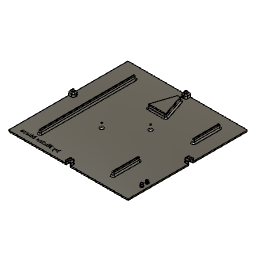
Wordclock_Backplate_Fusion360 (Autodesk Fusion 360 design; units mm, degrees)
Autodesk Fusion 360 part; units mm, degrees
(part 1 of 2)
sketch "Skizze3" plane through (0, 0, 0) normal (0, 0, 1) x (1, 0, 0)
  line L0 (0, 0) -> (204, 0)
  line L1 (204, 0) -> (204, 204)
  line L2 (204, 204) -> (0, 204)
  line L3 (0, 204) -> (0, 0)
  line L4 (2.15, 201.85) -> (201.85, 201.85)
  line L5 (201.85, 201.85) -> (201.85, 2.15)
  line L6 (201.85, 2.15) -> (2.15, 2.15)
  line L7 (2.15, 2.15) -> (2.15, 201.85)
  line L8 (98.5, 204) -> (105.5, 204)
  line L9 (105.5, 204) -> (105.5, 195)
  line L10 (105.5, 195) -> (98.5, 195)
  line L11 (98.5, 195) -> (98.5, 204)
  line L12 (0, 110.5) -> (9, 110.5)
  line L13 (9, 110.5) -> (9, 103.5)
  line L14 (9, 103.5) -> (0, 103.5)
  line L15 (0, 103.5) -> (0, 110.5)
  line L16 (204, 110.5) -> (195, 110.5)
  line L17 (195, 110.5) -> (195, 103.5)
  line L18 (195, 103.5) -> (204, 103.5)
  line L19 (204, 103.5) -> (204, 110.5)
  line L20 (0, 111.5) -> (10, 111.5)
  line L21 (10, 111.5) -> (10, 102.5)
  line L22 (10, 102.5) -> (0, 102.5)
  line L23 (0, 102.5) -> (0, 111.5)
  line L24 (204, 111.5) -> (194, 111.5)
  line L25 (194, 111.5) -> (194, 102.5)
  line L26 (194, 102.5) -> (204, 102.5)
  line L27 (204, 102.5) -> (204, 111.5)
  line L28 (97.5, 204) -> (106.5, 204)
  line L29 (106.5, 204) -> (106.5, 194)
  line L30 (106.5, 194) -> (97.5, 194)
  line L31 (97.5, 194) -> (97.5, 204)
  circle A0 centre (5.5, 107) radius 1.6
  circle A1 centre (102, 198.5) radius 1.6
  circle A2 centre (198.5, 107) radius 1.6
  line L32 (112, 184) -> (92, 184)
  line L33 (92, 184) -> (92, 154)
  line L34 (92, 154) -> (112, 154)
  line L35 (112, 154) -> (112, 184)
  line L36 (112, 154) -> (102, 184)
  line L37 (92, 154) -> (102, 184)
  line L38 (98.5, 0) -> (105.5, 0)
  line L39 (105.5, 0) -> (105.5, 9)
  line L40 (105.5, 9) -> (98.5, 9)
  line L41 (98.5, 9) -> (98.5, 0)
  line L42 (97.5, 0) -> (106.5, 0)
  line L43 (106.5, 0) -> (106.5, 10)
  line L44 (106.5, 10) -> (97.5, 10)
  line L45 (97.5, 10) -> (97.5, 0)
  circle A3 centre (102, 5.5) radius 1.6
  dimension "d16" = 204
  dimension "d17" = 204
  dimension "d18" = 2.15
  dimension "d19" = 2.15
  dimension "d20" = 2.15
  dimension "d21" = 2.15
  dimension "d22" = 7
  dimension "d23" = 9
  dimension "d24" = 98.5
  dimension "d25" = 9
  dimension "d26" = 7
  dimension "d27" = 93.5
  dimension "d28" = 9
  dimension "d29" = 7
  dimension "d30" = 93.5
  dimension "d35" = 1
  dimension "d36" = 1
  dimension "d37" = 1
  dimension "d38" = 1
  dimension "d39" = 1
  dimension "d40" = 1
  dimension "d41" = 1
  dimension "d42" = 1
  dimension "d43" = 1
  dimension "d54" = 3.2
  dimension "d55" = 3.5
  dimension "d56" = 5.5
  dimension "d57" = 3.2
  dimension "d58" = 5.5
  dimension "d59" = 3.5
  dimension "d60" = 3.2
  dimension "d61" = 3.5
  dimension "d62" = 5.5
  dimension "d65" = 20
  dimension "d66" = 30
  dimension "d67" = 20
  dimension "d68" = 92
  dimension "d168" = 7
  dimension "d169" = 9
  dimension "d170" = 98.5
  dimension "d171" = 1
  dimension "d172" = 1
  dimension "d173" = 1
  dimension "d174" = 3.2
  dimension "d175" = 3.5
  dimension "d176" = 5.5
  constraint horizontal L0
  constraint vertical L1
  constraint horizontal L2
  constraint vertical L3
  constraint coincident L0.start L3.end
  constraint horizontal L4
  constraint vertical L5
  constraint horizontal L6
  constraint vertical L7
  constraint horizontal L8
  constraint vertical L9
  constraint horizontal L10
  constraint vertical L11
  constraint coincident L2 L8.start
  constraint horizontal L12
  constraint vertical L13
  constraint horizontal L14
  constraint vertical L15
  constraint coincident L3 L12.start
  constraint horizontal L16
  constraint vertical L17
  constraint horizontal L18
  constraint vertical L19
  constraint coincident L1 L16.start
  constraint horizontal L20
  constraint vertical L21
  constraint horizontal L22
  constraint vertical L23
  constraint coincident L3 L20.start
  constraint horizontal L24
  constraint vertical L25
  constraint horizontal L26
  constraint vertical L27
  constraint coincident L1 L24.start
  constraint horizontal L28
  constraint vertical L29
  constraint horizontal L30
  constraint vertical L31
  constraint coincident L2 L28.start
  constraint horizontal L32
  constraint vertical L33
  constraint horizontal L34
  constraint vertical L35
  constraint midpoint L32 L36.end
  constraint horizontal L38
  constraint vertical L39
  constraint horizontal L40
  constraint vertical L41
  constraint coincident L0 L38.start
  constraint horizontal L42
  constraint vertical L43
  constraint horizontal L44
  constraint vertical L45
  constraint coincident L0 L42.start
  measures "d16" distance of L0.start L2.end
  measures "d17" distance of L0.start L0.end
  measures "d18" distance of L2 L4
  measures "d19" distance of L1 L5
  measures "d20" distance of L3 L7
  measures "d21" distance of L0 L6
  measures "d22" distance of L9.end L10.end
  measures "d23" distance of L8.start L10.end
  measures "d24" distance of L3 L11
  measures "d25" distance of L12.start L12.end
  measures "d26" distance of L12.end L13.end
  measures "d27" distance of L2 L12
  measures "d28" distance of L16.start L16.end
  measures "d29" distance of L16.end L17.end
  measures "d30" distance of L2 L16
  measures "d35" distance of L12 L20
  measures "d36" distance of L14 L22
  measures "d37" distance of L13 L21
  measures "d38" distance of L17 L25
  measures "d39" distance of L16 L24
  measures "d40" distance of L18 L26
  measures "d41" distance of L11 L31
  measures "d42" distance of L10 L30
  measures "d43" distance of L9 L29
  measures "d54" diameter of A0
  measures "d55" distance of L12 A0.centre
  measures "d56" distance of L23 A0.centre
  measures "d57" diameter of A1
  measures "d58" distance of L2 A1.centre
  measures "d59" distance of L9 A1.centre
  measures "d60" diameter of A2
  measures "d61" distance of L16 A2.centre
  measures "d62" distance of L1 A2.centre
  measures "d65" distance of L33.end L34.end
  measures "d66" distance of L32.start L34.end
  measures "d67" distance of L2 L32
  measures "d68" distance of L3 L33
  measures "d168" distance of L39.end L40.end
  measures "d169" distance of L38.start L40.end
  measures "d170" distance of L1 L39
  measures "d171" distance of L40 L44
  measures "d172" distance of L39 L43
  measures "d173" distance of L41 L45
  measures "d174" diameter of A3
  measures "d175" distance of L39 A3.centre
  measures "d176" distance of L0 A3.centre
extrude "Extrusion1" add sketch "Skizze3" along normal blind 2 contours L6 L39 L40 L41 L43 L44 L45 | L4 L5 L6 L7 L20 L21 L22 L24 L25 L26 L29 L30 L31 L43 L44 L45 | L6 L39 L40 L41 | L32 L35 L36 | L32 L33 L37 | L34 L36 L37 | A3
extrude "Extrusion2" add sketch "Skizze3" along normal blind 8 contours L6 L39 L40 L41 L43 L44 L45 | L7 L12 L13 L14 L20 L21 L22 | L6 L39 L40 L41 | L7 L12 L13 L14 | L5 L16 L17 L18 L24 L25 L26 | L4 L9 L10 L11 L29 L30 L31 | L5 L16 L17 L18 | L4 L9 L10 L11 | A0 | A1 | A2 | A3
fillet "Abrundung1" radius 1 4 edges at (201.85, 2.15, 1) (201.85, 201.85, 1) (2.15, 201.85, 1) (2.15, 2.15, 1)
extrude "Extrusion3" cut sketch "Skizze3" along normal blind 6 contours L6 L39 L40 L41 | L7 L12 L13 L14 | L5 L16 L17 L18 | L4 L9 L10 L11 | A0 | A1 | A2 | A3
fillet "Abrundung2" radius 3 8 edges at (194, 102.5, 5) (194, 111.5, 5) (97.5, 194, 5) (106.5, 194, 5) (106.5, 10, 5) (97.5, 10, 5) (10, 111.5, 5) (10, 102.5, 5)
extrude "Extrusion4" cut sketch "Skizze3" along normal blind 8 contours A0 | A1 | A2 | A3
extrude "Extrusion5" cut sketch "Skizze3" along normal blind 3 contours L34 L36 L37
sketch "Skizze4" plane through (0, 0, 2) normal (0, 0, 1) x (-1, 0, 0)
  line L0 (-112, -154) -> (-92, -154)
  line L1 (-92, -154) -> (-102, -184)
  line L2 (-102, -184) -> (-112, -154)
  line L3 (-2.15, -102.5) -> (-2.15, -3.15)
  arc A0 (-2.15, -3.15) -> (-3.15, -2.15) centre (-3.15, -3.15) ccw
  line L4 (-3.15, -2.15) -> (-97.5, -2.15)
  arc A1 (-200.85, -2.15) -> (-201.85, -3.15) centre (-200.85, -3.15) ccw
  line L5 (-201.85, -3.15) -> (-201.85, -102.5)
  arc A2 (-201.85, -200.85) -> (-200.85, -201.85) centre (-200.85, -200.85) ccw
  line L6 (-200.85, -201.85) -> (-106.5, -201.85)
  arc A3 (-3.15, -201.85) -> (-2.15, -200.85) centre (-3.15, -200.85) ccw
  line L7 (-2.15, -200.85) -> (-2.15, -111.5)
  line L8 (-89.2251, -152) -> (-115.201, -152)
  line L9 (-89.2147, -151.9686) -> (-100.633, -186.2236)
  line L10 (-103.3833, -186.1747) -> (-114.7974, -151.9325)
  line L11 (-104.7948, -188.2647) -> (-117.816, -149.2012)
  line L12 (-86.4032, -149.8589) -> (-99.2936, -188.5299)
  line L13 (-86, -150) -> (-118, -150)
  line L14 (-104, -186) -> (-100, -186)
  line L15 (-105.9099, -187.9999) -> (-98.0331, -188.0001)
  line L16 (-97.5, -2.15) -> (-97.5, -7)
  arc A4 (-100.5, -10) -> (-97.5, -7) centre (-100.5, -7) ccw
  line L17 (-100.5, -10) -> (-103.5, -10)
  arc A5 (-106.5, -7) -> (-103.5, -10) centre (-103.5, -7) ccw
  line L18 (-106.5, -7) -> (-106.5, -2.15)
  line L19 (-106.5, -2.15) -> (-200.85, -2.15)
  line L20 (-201.85, -102.5) -> (-197, -102.5)
  arc A6 (-194, -105.5) -> (-197, -102.5) centre (-197, -105.5) ccw
  line L21 (-194, -105.5) -> (-194, -108.5)
  arc A7 (-197, -111.5) -> (-194, -108.5) centre (-197, -108.5) ccw
  line L22 (-197, -111.5) -> (-201.85, -111.5)
  line L23 (-201.85, -111.5) -> (-201.85, -200.85)
  line L24 (-106.5, -201.85) -> (-106.5, -197)
  arc A8 (-103.5, -194) -> (-106.5, -197) centre (-103.5, -197) ccw
  line L25 (-103.5, -194) -> (-100.5, -194)
  arc A9 (-97.5, -197) -> (-100.5, -194) centre (-100.5, -197) ccw
  line L26 (-97.5, -197) -> (-97.5, -201.85)
  line L27 (-97.5, -201.85) -> (-3.15, -201.85)
  line L28 (-2.15, -111.5) -> (-7, -111.5)
  arc A10 (-10, -108.5) -> (-7, -111.5) centre (-7, -108.5) ccw
  line L29 (-10, -108.5) -> (-10, -105.5)
  arc A11 (-7, -102.5) -> (-10, -105.5) centre (-7, -105.5) ccw
  line L30 (-7, -102.5) -> (-2.15, -102.5)
  dimension "d75" = 2
  dimension "d78" = 2
  dimension "d79" = 2
  dimension "d84" = 2
  dimension "d85" = 2
  dimension "d86" = 2
  dimension "d87" = 2
  dimension "d88" = 2
  constraint horizontal L8
  constraint coincident L8.start L9
  constraint horizontal L13
  measures "d75" distance of L0 L8
  measures "d78" distance of L1 L9
  measures "d79" distance of L2 L10
  measures "d84" distance of L10 L11
  measures "d85" distance of L9 L12
  measures "d86" distance of L8 L13
  measures "d87" distance of L1.end L14
  measures "d88" distance of L14 L15
extrude "Extrusion8" add sketch "Skizze4" along normal blind 6.25 contours L11 L12 L13 L15
sketch "Skizze6" plane through (0, 0, 8.25) normal (0, 0, 1) x (-1, 0, 0)
  line L0 (-114.7749, -152) -> (-89.2251, -152)
  line L1 (-89.2251, -152) -> (-100.5585, -186)
  line L2 (-100.5585, -186) -> (-103.4415, -186)
  line L3 (-103.4415, -186) -> (-114.7749, -152)
  line L4 (-86.4503, -150) -> (-117.5497, -150)
  line L5 (-117.5497, -150) -> (-104.8831, -188)
  line L6 (-104.8831, -188) -> (-99.117, -188)
  line L7 (-99.117, -188) -> (-86.4503, -150)
extrude "Extrusion9" add sketch "Skizze6" against normal blind 2 contours L0 L1 L2 L3
fillet "Abrundung3" radius 2 3 edges at (102, 184, 1) (112, 154, 1) (92, 154, 1)
sketch "Skizze7" plane through (0, 0, 2) normal (0, 0, 1) x (-1, 0, 0)
  line L0 (-2.15, -102.5) -> (-2.15, -3.15)
  arc A0 (-2.15, -3.15) -> (-3.15, -2.15) centre (-3.15, -3.15) ccw
  line L1 (-3.15, -2.15) -> (-97.5, -2.15)
  arc A1 (-200.85, -2.15) -> (-201.85, -3.15) centre (-200.85, -3.15) ccw
  line L2 (-201.85, -3.15) -> (-201.85, -102.5)
  arc A2 (-201.85, -200.85) -> (-200.85, -201.85) centre (-200.85, -200.85) ccw
  line L3 (-200.85, -201.85) -> (-106.5, -201.85)
  arc A3 (-3.15, -201.85) -> (-2.15, -200.85) centre (-3.15, -200.85) ccw
  line L4 (-2.15, -200.85) -> (-2.15, -111.5)
  line L5 (-86.4503, -150) -> (-99.117, -188)
  line L6 (-99.117, -188) -> (-104.8831, -188)
  line L7 (-104.8831, -188) -> (-117.5497, -150)
  line L8 (-117.5497, -150) -> (-86.4503, -150)
  circle A4 centre (-77, -83) radius 1.25
  circle A5 centre (-120.538, -121.321) radius 1.25
  line L9 (-97.5, -2.15) -> (-97.5, -7)
  arc A6 (-100.5, -10) -> (-97.5, -7) centre (-100.5, -7) ccw
  line L10 (-100.5, -10) -> (-103.5, -10)
  arc A7 (-106.5, -7) -> (-103.5, -10) centre (-103.5, -7) ccw
  line L11 (-106.5, -7) -> (-106.5, -2.15)
  line L12 (-106.5, -2.15) -> (-200.85, -2.15)
  line L13 (-201.85, -102.5) -> (-197, -102.5)
  arc A8 (-194, -105.5) -> (-197, -102.5) centre (-197, -105.5) ccw
  line L14 (-194, -105.5) -> (-194, -108.5)
  arc A9 (-197, -111.5) -> (-194, -108.5) centre (-197, -108.5) ccw
  line L15 (-197, -111.5) -> (-201.85, -111.5)
  line L16 (-201.85, -111.5) -> (-201.85, -200.85)
  line L17 (-106.5, -201.85) -> (-106.5, -197)
  arc A10 (-103.5, -194) -> (-106.5, -197) centre (-103.5, -197) ccw
  line L18 (-103.5, -194) -> (-100.5, -194)
  arc A11 (-97.5, -197) -> (-100.5, -194) centre (-100.5, -197) ccw
  line L19 (-97.5, -197) -> (-97.5, -201.85)
  line L20 (-97.5, -201.85) -> (-3.15, -201.85)
  line L21 (-2.15, -111.5) -> (-7, -111.5)
  arc A12 (-10, -108.5) -> (-7, -111.5) centre (-7, -108.5) ccw
  line L22 (-10, -108.5) -> (-10, -105.5)
  arc A13 (-7, -102.5) -> (-10, -105.5) centre (-7, -105.5) ccw
  line L23 (-7, -102.5) -> (-2.15, -102.5)
  dimension "d95" = 2.5
  dimension "d97" = 74.85
  dimension "d98" = 2.5
  dimension "d99" = 80.529
  measures "d95" diameter of A4
  measures "d97" distance of L0 A4.centre
  measures "d98" diameter of A5
  measures "d99" distance of L3 A5.centre
extrude "Extrusion10" add sketch "Skizze7" along normal blind 8 contours A4 | A5
fillet "Abrundung4" radius 2 2 edges at (78.1654, 82.548, 2) (121.7034, 120.869, 2)
sketch "Skizze8" plane through (0, 0, 2) normal (0, 0, 1) x (-1, 0, 0)
  circle A0 centre (-77, -83) radius 3.25
  line L0 (-2.15, -102.5) -> (-2.15, -3.15)
  arc A1 (-2.15, -3.15) -> (-3.15, -2.15) centre (-3.15, -3.15) ccw
  line L1 (-3.15, -2.15) -> (-97.5, -2.15)
  arc A2 (-200.85, -2.15) -> (-201.85, -3.15) centre (-200.85, -3.15) ccw
  line L2 (-201.85, -3.15) -> (-201.85, -102.5)
  arc A3 (-201.85, -200.85) -> (-200.85, -201.85) centre (-200.85, -200.85) ccw
  line L3 (-200.85, -201.85) -> (-106.5, -201.85)
  arc A4 (-3.15, -201.85) -> (-2.15, -200.85) centre (-3.15, -200.85) ccw
  line L4 (-2.15, -200.85) -> (-2.15, -111.5)
  line L5 (-86.4503, -150) -> (-99.117, -188)
  line L6 (-99.117, -188) -> (-104.8831, -188)
  line L7 (-104.8831, -188) -> (-117.5497, -150)
  line L8 (-117.5497, -150) -> (-86.4503, -150)
  circle A5 centre (-120.538, -121.321) radius 3.25
  circle A6 centre (-194.85, -32.15) radius 2.5
  circle A7 centre (-194.85, -32.15) radius 1.5
  circle A8 centre (-194.85, -41.15) radius 2.5
  circle A9 centre (-194.85, -41.15) radius 1.5
  line L9 (-97.5, -2.15) -> (-97.5, -7)
  arc A10 (-100.5, -10) -> (-97.5, -7) centre (-100.5, -7) ccw
  line L10 (-100.5, -10) -> (-103.5, -10)
  arc A11 (-106.5, -7) -> (-103.5, -10) centre (-103.5, -7) ccw
  line L11 (-106.5, -7) -> (-106.5, -2.15)
  line L12 (-106.5, -2.15) -> (-200.85, -2.15)
  line L13 (-201.85, -102.5) -> (-197, -102.5)
  arc A12 (-194, -105.5) -> (-197, -102.5) centre (-197, -105.5) ccw
  line L14 (-194, -105.5) -> (-194, -108.5)
  arc A13 (-197, -111.5) -> (-194, -108.5) centre (-197, -108.5) ccw
  line L15 (-197, -111.5) -> (-201.85, -111.5)
  line L16 (-201.85, -111.5) -> (-201.85, -200.85)
  line L17 (-106.5, -201.85) -> (-106.5, -197)
  arc A14 (-103.5, -194) -> (-106.5, -197) centre (-103.5, -197) ccw
  line L18 (-103.5, -194) -> (-100.5, -194)
  arc A15 (-97.5, -197) -> (-100.5, -194) centre (-100.5, -197) ccw
  line L19 (-97.5, -197) -> (-97.5, -201.85)
  line L20 (-97.5, -201.85) -> (-3.15, -201.85)
  line L21 (-2.15, -111.5) -> (-7, -111.5)
  arc A16 (-10, -108.5) -> (-7, -111.5) centre (-7, -108.5) ccw
  line L22 (-10, -108.5) -> (-10, -105.5)
  arc A17 (-7, -102.5) -> (-10, -105.5) centre (-7, -105.5) ccw
  line L23 (-7, -102.5) -> (-2.15, -102.5)
  dimension "d105" = 5
  dimension "d106" = 7
  dimension "d107" = 30
  dimension "d108" = 3
  dimension "d109" = 5
  dimension "d110" = 3
  dimension "d111" = 7
  dimension "d112" = 9
  constraint concentric A6 A7
  constraint concentric A8 A9
  measures "d105" diameter of A6
  measures "d106" distance of L2 A6.centre
  measures "d107" distance of L1 A6.centre
  measures "d108" diameter of A7
  measures "d109" diameter of A8
  measures "d110" diameter of A9
  measures "d111" distance of L2 A8.centre
  measures "d112" distance of A6.centre A8.centre
extrude "Extrusion11" add sketch "Skizze8" along normal blind 1 contours A6 | A8
extrude "Extrusion12" add sketch "Skizze8" along normal blind 3.5 contours A7 | A9
sketch "Skizze9" plane through (0, 0, 5.5) normal (0, 0, 1) x (-1, 0, 0)
  circle A0 centre (-194.85, -41.15) radius 1.5
  circle A1 centre (-194.85, -41.15) radius 2
  circle A2 centre (-194.85, -32.15) radius 1.5
  circle A3 centre (-194.85, -32.15) radius 2
  dimension "d117" = 4
  dimension "d119" = 4
  constraint concentric A0 A1
  constraint concentric A2 A3
  measures "d117" diameter of A1
  measures "d119" diameter of A3
extrude "Extrusion13" add sketch "Skizze9" along normal blind 2 contours A0 | A1 | A2 | A3
sketch "Skizze10" plane through (0, 0, 7.5) normal (0, 0, 1) x (-1, 0, 0)
  circle A0 centre (-194.85, -41.15) radius 2
  line L0 (-193.1, -42.9) -> (-196.6, -42.9)
  line L1 (-196.6, -42.9) -> (-196.6, -39.4)
  line L2 (-196.6, -39.4) -> (-193.1, -39.4)
  line L3 (-193.1, -39.4) -> (-193.1, -42.9)
  line L4 (-193.1, -42.9) -> (-196.6, -39.4)
  line L5 (-192.7464, -42.5464) -> (-196.2464, -39.0464)
  line L6 (-193.4667, -43.2404) -> (-196.9667, -39.7404)
  line L7 (-193.1, -30.4) -> (-193.1, -33.9)
  line L8 (-192.7596, -30.7667) -> (-196.2596, -34.2667)
  line L9 (-193.1, -30.4) -> (-196.6, -33.9)
  line L10 (-193.4536, -30.0464) -> (-196.9536, -33.5464)
  line L11 (-196.6, -30.4) -> (-193.1, -30.4)
  line L12 (-196.6, -33.9) -> (-196.6, -30.4)
  line L13 (-193.1, -33.9) -> (-196.6, -33.9)
  dimension "d122" = 1.75
  dimension "d123" = 3.5
  dimension "d124" = 1.75
  dimension "d125" = 3.5
  dimension "d127" = 1
  dimension "d128" = 0.5
  dimension "d129" = 3.5
  dimension "d130" = 3.5
  dimension "d131" = 1
  dimension "d132" = 0.5
  constraint horizontal L0
  constraint vertical L1
  constraint horizontal L2
  constraint vertical L3
  measures "d122" distance of A0.centre L3
  measures "d123" distance of L1 L3
  measures "d124" distance of A0.centre L0
  measures "d125" distance of L0.end L1.end
  measures "d127" distance of L5 L6
  measures "d128" distance of L4 L5
  measures "d129" distance of L11 L13
  measures "d130" distance of L7.end L9.end
  measures "d131" distance of L8 L10
  measures "d132" distance of L9 L10
chamfer "Fase1" distance 1.5 angle 45 2 edges at (196.7147, 41.8732, 7.5) (196.7147, 32.8732, 7.5)
extrude "Extrusion14" cut sketch "Skizze10" against normal blind 5 contours A0 L3 L4 L5 | A0 L4 L5 | A0 L0 L4 L6 | A0 L4 L6 | A0 L2 L4 L5 | A0 L1 L4 L6 | L7 L8 L9 L13 | L9 L10 L11 L12
fillet "Abrundung10" radius 3 8 edges at (98.5, 195, 3) (105.5, 195, 3) (9, 103.5, 3) (9, 110.5, 3) (105.5, 9, 3) (98.5, 9, 3) (195, 110.5, 3) (195, 103.5, 3)
fillet "Abrundung11" radius 2 20 edges at (4.575, 102.5, 8) (9.1213, 103.3787, 8) (10, 107, 8) (9.1213, 110.6213, 8) (4.575, 111.5, 8) (106.5, 199.425, 8) (105.6213, 194.8787, 8) (102, 194, 8) (98.3787, 194.8787, 8) (97.5, 199.425, 8) (199.425, 102.5, 8) (194.8787, 103.3787, 8) (194, 107, 8) (194.8787, 110.6213, 8) (199.425, 111.5, 8) (106.5, 4.575, 8) (105.6213, 9.1213, 8) (102, 10, 8) (98.3787, 9.1213, 8) (97.5, 4.575, 8)
sketch "Skizze11" plane through (0, 0, 2) normal (0, 0, 1) x (-1, 0, 0)
  circle A0 centre (-194.85, -41.15) radius 2.5
  circle A1 centre (-77, -83) radius 3.25
  line L0 (-2.15, -102.5) -> (-2.15, -3.15)
  arc A2 (-2.15, -3.15) -> (-3.15, -2.15) centre (-3.15, -3.15) ccw
  line L1 (-3.15, -2.15) -> (-97.5, -2.15)
  arc A3 (-200.85, -2.15) -> (-201.85, -3.15) centre (-200.85, -3.15) ccw
  line L2 (-201.85, -3.15) -> (-201.85, -102.5)
  arc A4 (-201.85, -200.85) -> (-200.85, -201.85) centre (-200.85, -200.85) ccw
  line L3 (-200.85, -201.85) -> (-106.5, -201.85)
  arc A5 (-3.15, -201.85) -> (-2.15, -200.85) centre (-3.15, -200.85) ccw
  line L4 (-2.15, -200.85) -> (-2.15, -111.5)
  line L5 (-86.4503, -150) -> (-99.117, -188)
  line L6 (-99.117, -188) -> (-104.8831, -188)
  line L7 (-104.8831, -188) -> (-117.5497, -150)
  line L8 (-117.5497, -150) -> (-86.4503, -150)
  circle A6 centre (-120.538, -121.321) radius 3.25
  circle A7 centre (-194.85, -32.15) radius 2.5
  line L9 (-32.15, -181.85) -> (-35.15, -181.85)
  line L10 (-35.15, -181.85) -> (-35.15, -22.15)
  line L11 (-35.15, -22.15) -> (-32.15, -22.15)
  line L12 (-32.15, -22.15) -> (-32.15, -181.85)
  line L13 (-173.85, -181.85) -> (-176.85, -181.85)
  line L14 (-176.85, -181.85) -> (-176.85, -136.85)
  line L15 (-176.85, -136.85) -> (-173.85, -136.85)
  line L16 (-173.85, -136.85) -> (-173.85, -181.85)
  line L17 (-153.85, -67.15) -> (-156.85, -67.15)
  line L18 (-156.85, -67.15) -> (-156.85, -22.15)
  line L19 (-156.85, -22.15) -> (-153.85, -22.15)
  line L20 (-153.85, -22.15) -> (-153.85, -67.15)
  line L21 (-97.5, -2.15) -> (-97.5, -7)
  arc A8 (-100.5, -10) -> (-97.5, -7) centre (-100.5, -7) ccw
  line L22 (-100.5, -10) -> (-103.5, -10)
  arc A9 (-106.5, -7) -> (-103.5, -10) centre (-103.5, -7) ccw
  line L23 (-106.5, -7) -> (-106.5, -2.15)
  line L24 (-106.5, -2.15) -> (-200.85, -2.15)
  line L25 (-201.85, -102.5) -> (-197, -102.5)
  arc A10 (-194, -105.5) -> (-197, -102.5) centre (-197, -105.5) ccw
  line L26 (-194, -105.5) -> (-194, -108.5)
  arc A11 (-197, -111.5) -> (-194, -108.5) centre (-197, -108.5) ccw
  line L27 (-197, -111.5) -> (-201.85, -111.5)
  line L28 (-201.85, -111.5) -> (-201.85, -200.85)
  line L29 (-106.5, -201.85) -> (-106.5, -197)
  arc A12 (-103.5, -194) -> (-106.5, -197) centre (-103.5, -197) ccw
  line L30 (-103.5, -194) -> (-100.5, -194)
  arc A13 (-97.5, -197) -> (-100.5, -194) centre (-100.5, -197) ccw
  line L31 (-97.5, -197) -> (-97.5, -201.85)
  line L32 (-97.5, -201.85) -> (-3.15, -201.85)
  line L33 (-2.15, -111.5) -> (-7, -111.5)
  arc A14 (-10, -108.5) -> (-7, -111.5) centre (-7, -108.5) ccw
  line L34 (-10, -108.5) -> (-10, -105.5)
  arc A15 (-7, -102.5) -> (-10, -105.5) centre (-7, -105.5) ccw
  line L35 (-7, -102.5) -> (-2.15, -102.5)
  dimension "d136" = 3
  dimension "d138" = 20
  dimension "d139" = 20
  dimension "d145" = 45
  dimension "d147" = 3
  dimension "d149" = 3
  dimension "d150" = 45
  dimension "d151" = 20
  dimension "d152" = 30
  dimension "d154" = 45
  dimension "d181" = 25
  constraint horizontal L9
  constraint vertical L10
  constraint horizontal L11
  constraint vertical L12
  constraint horizontal L13
  constraint vertical L14
  constraint horizontal L15
  constraint vertical L16
  constraint horizontal L17
  constraint vertical L18
  constraint horizontal L19
  constraint vertical L20
  measures "d136" distance of L10 L12
  measures "d138" distance of L3 L9
  measures "d139" distance of L1 L11
  measures "d145" distance of L13.end L14.end
  measures "d147" distance of L13.start L13.end
  measures "d149" distance of L17.start L17.end
  measures "d150" distance of L17.end L18.end
  measures "d151" distance of L1 L19
  measures "d152" distance of L4 L12
  measures "d154" distance of L2 L18
  measures "d181" distance of L14 L28
extrude "Extrusion16" add sketch "Skizze11" along normal blind 6.25 contours L9 L10 L11 L12 | L13 L14 L15 L16 | L17 L18 L19 L20
sketch "Skizze12" plane through (0, 0, 0) normal (0, 0, -1) x (1, 0, 0)
  line L0 (94.7749, -154) -> (109.2251, -154)
  arc A0 (111.1225, -156.6325) -> (109.2251, -154) centre (109.2251, -156) ccw
  line L1 (111.1225, -156.6325) -> (103.8974, -178.3079)
  arc A1 (100.1026, -178.3079) -> (103.8974, -178.3079) centre (102, -177.6754) ccw
  line L2 (100.1026, -178.3079) -> (92.8775, -156.6325)
  arc A2 (94.7749, -154) -> (92.8775, -156.6325) centre (94.7749, -156) ccw
  line L3 (6, -110.5) -> (2.15, -110.5)
  line L4 (2.15, -110.5) -> (2.15, -200.85)
  arc A3 (2.15, -200.85) -> (3.15, -201.85) centre (3.15, -200.85) ccw
  line L5 (3.15, -201.85) -> (98.5, -201.85)
  line L6 (98.5, -201.85) -> (98.5, -198)
  line L7 (101.5, -195) -> (102.5, -195)
  line L8 (105.5, -198) -> (105.5, -201.85)
  line L9 (105.5, -201.85) -> (200.85, -201.85)
  arc A4 (200.85, -201.85) -> (201.85, -200.85) centre (200.85, -200.85) ccw
  line L10 (201.85, -200.85) -> (201.85, -110.5)
  line L11 (201.85, -110.5) -> (198, -110.5)
  line L12 (195, -107.5) -> (195, -106.5)
  line L13 (198, -103.5) -> (201.85, -103.5)
  line L14 (201.85, -103.5) -> (201.85, -3.15)
  arc A5 (201.85, -3.15) -> (200.85, -2.15) centre (200.85, -3.15) ccw
  line L15 (200.85, -2.15) -> (105.5, -2.15)
  arc A6 (3.15, -2.15) -> (2.15, -3.15) centre (3.15, -3.15) ccw
  line L16 (2.15, -3.15) -> (2.15, -103.5)
  line L17 (2.15, -103.5) -> (6, -103.5)
  line L18 (9, -106.5) -> (9, -107.5)
  line L19 (75.219, -11.0615) -> (75.219, -11.7939)
  line L20 (75.219, -11.7939) -> (74.4736, -11.7939)
  line L21 (74.4736, -11.7939) -> (74.4736, -16.3578)
  line L22 (74.4736, -16.3578) -> (75.219, -16.3578)
  line L23 (75.219, -16.3578) -> (75.219, -17.0903)
  line L24 (75.219, -17.0903) -> (73.6674, -17.0903)
  line L25 (73.6674, -17.0903) -> (73.6674, -14.6631)
  spline S0 degree 2 poles (73.6674, -14.6631) (73.0476, -15.3739) (72.1461, -15.3739) knots 0 0 0 1 1 1
  spline S1 degree 2 poles (72.1461, -15.3739) (71.2793, -15.3739) (70.6942, -14.7758) knots 0 0 0 1 1 1
  spline S2 degree 2 poles (70.6942, -14.7758) (70.1047, -14.1821) (70.1047, -13.2069) knots 0 0 0 1 1 1
  spline S3 degree 2 poles (70.1047, -13.2069) (70.1047, -12.2707) (70.6812, -11.6292) knots 0 0 0 1 1 1
  spline S4 degree 2 poles (70.6812, -11.6292) (71.2533, -10.9921) (72.1504, -10.9921) knots 0 0 0 1 1 1
  spline S5 degree 2 poles (72.1504, -10.9921) (72.6532, -10.9921) (73.0693, -11.2088) knots 0 0 0 1 1 1
  spline S6 degree 2 poles (73.0693, -11.2088) (73.4854, -11.4255) (73.6674, -11.6899) knots 0 0 0 1 1 1
  line L26 (73.6674, -11.6899) -> (73.6674, -11.0615)
  line L27 (73.6674, -11.0615) -> (75.219, -11.0615)
  spline S7 degree 2 poles (73.6414, -13.1505) (73.6414, -12.4961) (73.2426, -12.1103) knots 0 0 0 1 1 1
  spline S8 degree 2 poles (73.2426, -12.1103) (72.8396, -11.7289) (72.3151, -11.7289) knots 0 0 0 1 1 1
  spline S9 degree 2 poles (72.3151, -11.7289) (71.7647, -11.7289) (71.366, -12.1363) knots 0 0 0 1 1 1
  spline S10 degree 2 poles (71.366, -12.1363) (70.9672, -12.5437) (70.9672, -13.2285) knots 0 0 0 1 1 1
  spline S11 degree 2 poles (70.9672, -13.2285) (70.9672, -13.8917) (71.366, -14.2557) knots 0 0 0 1 1 1
  spline S12 degree 2 poles (71.366, -14.2557) (71.7604, -14.6241) (72.2935, -14.6241) knots 0 0 0 1 1 1
  spline S13 degree 2 poles (72.2935, -14.6241) (72.8179, -14.6241) (73.2296, -14.2427) knots 0 0 0 1 1 1
  spline S14 degree 2 poles (73.2296, -14.2427) (73.6414, -13.8657) (73.6414, -13.1505) knots 0 0 0 1 1 1
  line L28 (67.916, -11.1351) -> (69.2942, -14.5244)
  line L29 (69.2942, -14.5244) -> (69.992, -14.5244)
  line L30 (69.992, -14.5244) -> (69.992, -15.2569)
  line L31 (69.992, -15.2569) -> (67.916, -15.2569)
  line L32 (67.916, -15.2569) -> (67.916, -14.5244)
  line L33 (67.916, -14.5244) -> (68.4187, -14.5244)
  line L34 (68.4187, -14.5244) -> (67.5129, -12.2013)
  line L35 (67.5129, -12.2013) -> (66.6244, -14.5244)
  line L36 (66.6244, -14.5244) -> (67.1792, -14.5244)
  line L37 (67.1792, -14.5244) -> (67.1792, -15.2569)
  line L38 (67.1792, -15.2569) -> (65.1464, -15.2569)
  line L39 (65.1464, -15.2569) -> (65.1464, -14.5244)
  line L40 (65.1464, -14.5244) -> (65.7706, -14.5244)
  line L41 (65.7706, -14.5244) -> (67.8466, -9.1804)
  line L42 (67.8466, -9.1804) -> (69.2379, -9.1804)
  line L43 (69.2379, -9.1804) -> (69.2379, -9.8999)
  line L44 (69.2379, -9.8999) -> (68.4187, -9.8999)
  line L45 (68.4187, -9.8999) -> (67.916, -11.1351)
  line L46 (61.9435, -11.8156) -> (61.9435, -16.3361)
  line L47 (61.9435, -16.3361) -> (62.806, -16.3361)
  line L48 (62.806, -16.3361) -> (62.806, -17.0903)
  line L49 (62.806, -17.0903) -> (60.7473, -17.0903)
  line L50 (60.7473, -17.0903) -> (58.1034, -12.405)
  line L51 (58.1034, -12.405) -> (58.1034, -16.3361)
  line L52 (58.1034, -16.3361) -> (58.9573, -16.3361)
  line L53 (58.9573, -16.3361) -> (58.9573, -17.0903)
  line L54 (58.9573, -17.0903) -> (56.4825, -17.0903)
  line L55 (56.4825, -17.0903) -> (56.4825, -16.3361)
  line L56 (56.4825, -16.3361) -> (57.371, -16.3361)
  line L57 (57.371, -16.3361) -> (57.371, -11.0008)
  line L58 (57.371, -11.0008) -> (58.3072, -11.0008)
  line L59 (58.3072, -11.0008) -> (61.198, -16.1454)
  line L60 (61.198, -16.1454) -> (61.198, -11.8156)
  line L61 (61.198, -11.8156) -> (60.3355, -11.8156)
  line L62 (60.3355, -11.8156) -> (60.3355, -11.0614)
  line L63 (60.3355, -11.0614) -> (62.806, -11.0614)
  line L64 (62.806, -11.0614) -> (62.806, -11.8156)
  line L65 (62.806, -11.8156) -> (61.9435, -11.8156)
  spline S15 degree 2 poles (55.646, -16.6829) (55.646, -16.8822) (55.5073, -17.0296) knots 0 0 0 1 1 1
  spline S16 degree 2 poles (55.5073, -17.0296) (55.3643, -17.1769) (55.1476, -17.1769) knots 0 0 0 1 1 1
  spline S17 degree 2 poles (55.1476, -17.1769) (54.9438, -17.1769) (54.7965, -17.0339) knots 0 0 0 1 1 1
  spline S18 degree 2 poles (54.7965, -17.0339) (54.6491, -16.8909) (54.6491, -16.6829) knots 0 0 0 1 1 1
  spline S19 degree 2 poles (54.6491, -16.6829) (54.6491, -16.4748) (54.7965, -16.3275) knots 0 0 0 1 1 1
  spline S20 degree 2 poles (54.7965, -16.3275) (54.9438, -16.1844) (55.1476, -16.1844) knots 0 0 0 1 1 1
  spline S21 degree 2 poles (55.1476, -16.1844) (55.3556, -16.1844) (55.503, -16.3318) knots 0 0 0 1 1 1
  spline S22 degree 2 poles (55.503, -16.3318) (55.646, -16.4791) (55.646, -16.6829) knots 0 0 0 1 1 1
  line L66 (55.529, -11.7939) -> (55.529, -14.5244)
  line L67 (55.529, -14.5244) -> (56.1834, -14.5244)
  line L68 (56.1834, -14.5244) -> (56.1834, -15.2569)
  line L69 (56.1834, -15.2569) -> (54.7055, -15.2569)
  line L70 (54.7055, -15.2569) -> (54.7055, -11.7939)
  line L71 (54.7055, -11.7939) -> (54.0597, -11.7939)
  line L72 (54.0597, -11.7939) -> (54.0597, -11.0615)
  line L73 (54.0597, -11.0615) -> (56.1834, -11.0615)
  line L74 (56.1834, -11.0615) -> (56.1834, -11.7939)
  line L75 (56.1834, -11.7939) -> (55.529, -11.7939)
  line L76 (49.5782, -15.2569) -> (49.5782, -13.6706)
  line L77 (49.5782, -13.6706) -> (50.315, -13.6706)
  spline S23 degree 2 poles (50.315, -13.6706) (50.3713, -14.1257) (50.6877, -14.3684) knots 0 0 0 1 1 1
  spline S24 degree 2 poles (50.6877, -14.3684) (50.9998, -14.6111) (51.4158, -14.6111) knots 0 0 0 1 1 1
  spline S25 degree 2 poles (51.4158, -14.6111) (51.9706, -14.6111) (52.3174, -14.2167) knots 0 0 0 1 1 1
  spline S26 degree 2 poles (52.3174, -14.2167) (52.6641, -13.8267) (52.6641, -13.1895) knots 0 0 0 1 1 1
  spline S27 degree 2 poles (52.6641, -13.1895) (52.6641, -12.5958) (52.3347, -12.1407) knots 0 0 0 1 1 1
  spline S28 degree 2 poles (52.3347, -12.1407) (52.0053, -11.6899) (51.3812, -11.6899) knots 0 0 0 1 1 1
  spline S29 degree 2 poles (51.3812, -11.6899) (50.5143, -11.6899) (50.1243, -12.5134) knots 0 0 0 1 1 1
  line L78 (50.1243, -12.5134) -> (49.4438, -12.1927)
  spline S30 degree 2 poles (49.4438, -12.1927) (50.0072, -10.9401) (51.4158, -10.9401) knots 0 0 0 1 1 1
  spline S31 degree 2 poles (51.4158, -10.9401) (52.4127, -10.9401) (52.9848, -11.6206) knots 0 0 0 1 1 1
  spline S32 degree 2 poles (52.9848, -11.6206) (53.5569, -12.301) (53.5569, -13.1895) knots 0 0 0 1 1 1
  spline S33 degree 2 poles (53.5569, -13.1895) (53.5569, -14.1387) (52.9328, -14.7542) knots 0 0 0 1 1 1
  spline S34 degree 2 poles (52.9328, -14.7542) (52.3087, -15.3739) (51.4939, -15.3739) knots 0 0 0 1 1 1
  spline S35 degree 2 poles (51.4939, -15.3739) (50.7961, -15.3739) (50.315, -14.9622) knots 0 0 0 1 1 1
  line L79 (50.315, -14.9622) -> (50.315, -15.2569)
  line L80 (50.315, -15.2569) -> (49.5782, -15.2569)
  line L81 (48.3169, -11.7939) -> (48.3169, -16.3578)
  line L82 (48.3169, -16.3578) -> (49.0624, -16.3578)
  line L83 (49.0624, -16.3578) -> (49.0624, -17.0903)
  line L84 (49.0624, -17.0903) -> (47.4934, -17.0903)
  line L85 (47.4934, -17.0903) -> (47.4934, -11.7939)
  line L86 (47.4934, -11.7939) -> (46.852, -11.7939)
  line L87 (46.852, -11.7939) -> (46.852, -11.0615)
  line L88 (46.852, -11.0615) -> (49.0624, -11.0615)
  line L89 (49.0624, -11.0615) -> (49.0624, -11.7939)
  line L90 (49.0624, -11.7939) -> (48.3169, -11.7939)
  line L91 (42.0411, -11.7939) -> (42.0411, -11.0615)
  line L92 (42.0411, -11.0615) -> (43.48, -11.0615)
  line L93 (43.48, -11.0615) -> (43.48, -11.5729)
  spline S36 degree 2 poles (43.48, -11.5729) (44.0781, -10.9921) (44.8149, -10.9921) knots 0 0 0 1 1 1
  spline S37 degree 2 poles (44.8149, -10.9921) (45.387, -10.9921) (45.8118, -11.3648) knots 0 0 0 1 1 1
  spline S38 degree 2 poles (45.8118, -11.3648) (46.2322, -11.7376) (46.2322, -12.3184) knots 0 0 0 1 1 1
  spline S39 degree 2 poles (46.2322, -12.3184) (46.2322, -12.9035) (45.7858, -13.2892) knots 0 0 0 1 1 1
  spline S40 degree 2 poles (45.7858, -13.2892) (45.335, -13.675) (44.7022, -13.675) knots 0 0 0 1 1 1
  spline S41 degree 2 poles (44.7022, -13.675) (44.1128, -13.675) (43.5624, -13.3196) knots 0 0 0 1 1 1
  line L94 (43.5624, -13.3196) -> (43.5624, -13.7356)
  spline S42 degree 2 poles (43.5624, -13.7356) (43.5624, -14.0564) (43.623, -14.2297) knots 0 0 0 1 1 1
  spline S43 degree 2 poles (43.623, -14.2297) (43.6837, -14.4031) (43.9091, -14.5418) knots 0 0 0 1 1 1
  spline S44 degree 2 poles (43.9091, -14.5418) (44.1301, -14.6805) (44.4898, -14.6805) knots 0 0 0 1 1 1
  spline S45 degree 2 poles (44.4898, -14.6805) (45.1096, -14.6805) (45.387, -14.1864) knots 0 0 0 1 1 1
  line L95 (45.387, -14.1864) -> (46.1758, -14.3944)
  spline S46 degree 2 poles (46.1758, -14.3944) (45.6514, -15.3739) (44.3642, -15.3739) knots 0 0 0 1 1 1
  spline S47 degree 2 poles (44.3642, -15.3739) (43.8917, -15.3739) (43.5493, -15.2439) knots 0 0 0 1 1 1
  spline S48 degree 2 poles (43.5493, -15.2439) (43.2026, -15.1182) (43.0336, -14.9145) knots 0 0 0 1 1 1
  spline S49 degree 2 poles (43.0336, -14.9145) (42.8645, -14.7152) (42.8082, -14.4811) knots 0 0 0 1 1 1
  spline S50 degree 2 poles (42.8082, -14.4811) (42.7475, -14.2471) (42.7475, -13.7356) knots 0 0 0 1 1 1
  line L96 (42.7475, -13.7356) -> (42.7475, -11.7939)
  line L97 (42.7475, -11.7939) -> (42.0411, -11.7939)
  spline S51 degree 2 poles (43.5624, -12.6217) (44.0955, -13.0378) (44.6416, -13.0378) knots 0 0 0 1 1 1
  spline S52 degree 2 poles (44.6416, -13.0378) (44.984, -13.0378) (45.2137, -12.8385) knots 0 0 0 1 1 1
  spline S53 degree 2 poles (45.2137, -12.8385) (45.4434, -12.6391) (45.4434, -12.3227) knots 0 0 0 1 1 1
  spline S54 degree 2 poles (45.4434, -12.3227) (45.4434, -12.028) (45.244, -11.8286) knots 0 0 0 1 1 1
  spline S55 degree 2 poles (45.244, -11.8286) (45.0403, -11.6292) (44.6936, -11.6292) knots 0 0 0 1 1 1
  spline S56 degree 2 poles (44.6936, -11.6292) (44.0955, -11.6292) (43.5624, -12.132) knots 0 0 0 1 1 1
  line L98 (43.5624, -12.132) -> (43.5624, -12.6217)
  line L99 (41.56, -11.0615) -> (41.56, -12.5004)
  line L100 (41.56, -12.5004) -> (40.8232, -12.5004)
  line L101 (40.8232, -12.5004) -> (40.8232, -12.3617)
  spline S57 degree 2 poles (40.8232, -12.3617) (40.7842, -12.067) (40.5068, -11.8763) knots 0 0 0 1 1 1
  spline S58 degree 2 poles (40.5068, -11.8763) (40.2251, -11.6856) (39.8437, -11.6856) knots 0 0 0 1 1 1
  spline S59 degree 2 poles (39.8437, -11.6856) (39.4449, -11.6856) (39.2065, -11.8243) knots 0 0 0 1 1 1
  spline S60 degree 2 poles (39.2065, -11.8243) (38.9682, -11.963) (38.9682, -12.21) knots 0 0 0 1 1 1
  spline S61 degree 2 poles (38.9682, -12.21) (38.9682, -12.4484) (39.1675, -12.5611) knots 0 0 0 1 1 1
  spline S62 degree 2 poles (39.1675, -12.5611) (39.3626, -12.6738) (39.9477, -12.7691) knots 0 0 0 1 1 1
  spline S63 degree 2 poles (39.9477, -12.7691) (40.8145, -12.9165) (41.1872, -13.2415) knots 0 0 0 1 1 1
  spline S64 degree 2 poles (41.1872, -13.2415) (41.5556, -13.5709) (41.5556, -14.091) knots 0 0 0 1 1 1
  spline S65 degree 2 poles (41.5556, -14.091) (41.5556, -14.6155) (41.1526, -14.9665) knots 0 0 0 1 1 1
  spline S66 degree 2 poles (41.1526, -14.9665) (40.7495, -15.3219) (40.0907, -15.3219) knots 0 0 0 1 1 1
  spline S67 degree 2 poles (40.0907, -15.3219) (39.4969, -15.3219) (39.0678, -15.0792) knots 0 0 0 1 1 1
  line L102 (39.0678, -15.0792) -> (39.0678, -15.2569)
  line L103 (39.0678, -15.2569) -> (38.3354, -15.2569)
  line L104 (38.3354, -15.2569) -> (38.3354, -13.8657)
  line L105 (38.3354, -13.8657) -> (39.0678, -13.8657)
  line L106 (39.0678, -13.8657) -> (39.0678, -14.1214)
  spline S68 degree 2 poles (39.0678, -14.1214) (39.4016, -14.6371) (40.0387, -14.6371) knots 0 0 0 1 1 1
  spline S69 degree 2 poles (40.0387, -14.6371) (40.3638, -14.6371) (40.5761, -14.4941) knots 0 0 0 1 1 1
  spline S70 degree 2 poles (40.5761, -14.4941) (40.7842, -14.3554) (40.7842, -14.1214) knots 0 0 0 1 1 1
  spline S71 degree 2 poles (40.7842, -14.1214) (40.7842, -13.883) (40.5935, -13.792) knots 0 0 0 1 1 1
  spline S72 degree 2 poles (40.5935, -13.792) (40.3984, -13.7053) (39.7613, -13.6056) knots 0 0 0 1 1 1
  spline S73 degree 2 poles (39.7613, -13.6056) (39.1502, -13.5103) (38.8381, -13.3802) knots 0 0 0 1 1 1
  spline S74 degree 2 poles (38.8381, -13.3802) (38.5261, -13.2545) (38.3224, -12.9555) knots 0 0 0 1 1 1
  spline S75 degree 2 poles (38.3224, -12.9555) (38.1143, -12.6608) (38.1143, -12.2664) knots 0 0 0 1 1 1
  spline S76 degree 2 poles (38.1143, -12.2664) (38.1143, -11.6812) (38.5651, -11.3345) knots 0 0 0 1 1 1
  spline S77 degree 2 poles (38.5651, -11.3345) (39.0115, -10.9921) (39.7266, -10.9921) knots 0 0 0 1 1 1
  spline S78 degree 2 poles (39.7266, -10.9921) (40.3984, -10.9921) (40.8232, -11.2955) knots 0 0 0 1 1 1
  line L107 (40.8232, -11.2955) -> (40.8232, -11.0615)
  line L108 (40.8232, -11.0615) -> (41.56, -11.0615)
  line L109 (34.6903, -11.8156) -> (34.6903, -16.3361)
  line L110 (34.6903, -16.3361) -> (35.4142, -16.3361)
  line L111 (35.4142, -16.3361) -> (35.4142, -17.0903)
  line L112 (35.4142, -17.0903) -> (33.3511, -17.0903)
  line L113 (33.3511, -17.0903) -> (31.7648, -12.9598)
  line L114 (31.7648, -12.9598) -> (30.1612, -17.0903)
  line L115 (30.1612, -17.0903) -> (28.0764, -17.0903)
  line L116 (28.0764, -17.0903) -> (28.0764, -16.3361)
  line L117 (28.0764, -16.3361) -> (28.8046, -16.3361)
  line L118 (28.8046, -16.3361) -> (28.8046, -11.8156)
  line L119 (28.8046, -11.8156) -> (28.0764, -11.8156)
  line L120 (28.0764, -11.8156) -> (28.0764, -11.0615)
  line L121 (28.0764, -11.0615) -> (30.3475, -11.0615)
  line L122 (30.3475, -11.0615) -> (30.3475, -11.8156)
  line L123 (30.3475, -11.8156) -> (29.628, -11.8156)
  line L124 (29.628, -11.8156) -> (29.628, -16.3361)
  line L125 (29.628, -16.3361) -> (31.7084, -11.0008)
  line L126 (31.7084, -11.0008) -> (31.8862, -11.0008)
  line L127 (31.8862, -11.0008) -> (33.9449, -16.3361)
  line L128 (33.9449, -16.3361) -> (33.9449, -11.8156)
  line L129 (33.9449, -11.8156) -> (33.2817, -11.8156)
  line L130 (33.2817, -11.8156) -> (33.2817, -11.0615)
  line L131 (33.2817, -11.0615) -> (35.4142, -11.0615)
  line L132 (35.4142, -11.0615) -> (35.4142, -11.8156)
  line L133 (35.4142, -11.8156) -> (34.6903, -11.8156)
  spline S79 degree 2 poles (27.0406, -16.6829) (27.0406, -16.8822) (26.9019, -17.0296) knots 0 0 0 1 1 1
  spline S80 degree 2 poles (26.9019, -17.0296) (26.7588, -17.1769) (26.5421, -17.1769) knots 0 0 0 1 1 1
  spline S81 degree 2 poles (26.5421, -17.1769) (26.3384, -17.1769) (26.1911, -17.0339) knots 0 0 0 1 1 1
  spline S82 degree 2 poles (26.1911, -17.0339) (26.0437, -16.8909) (26.0437, -16.6829) knots 0 0 0 1 1 1
  spline S83 degree 2 poles (26.0437, -16.6829) (26.0437, -16.4748) (26.1911, -16.3275) knots 0 0 0 1 1 1
  spline S84 degree 2 poles (26.1911, -16.3275) (26.3384, -16.1844) (26.5421, -16.1844) knots 0 0 0 1 1 1
  spline S85 degree 2 poles (26.5421, -16.1844) (26.7502, -16.1844) (26.8975, -16.3318) knots 0 0 0 1 1 1
  spline S86 degree 2 poles (26.8975, -16.3318) (27.0406, -16.4791) (27.0406, -16.6829) knots 0 0 0 1 1 1
  line L134 (26.9235, -11.7939) -> (26.9235, -14.5244)
  line L135 (26.9235, -14.5244) -> (27.578, -14.5244)
  line L136 (27.578, -14.5244) -> (27.578, -15.2569)
  line L137 (27.578, -15.2569) -> (26.1, -15.2569)
  line L138 (26.1, -15.2569) -> (26.1, -11.7939)
  line L139 (26.1, -11.7939) -> (25.4543, -11.7939)
  line L140 (25.4543, -11.7939) -> (25.4543, -11.0615)
  line L141 (25.4543, -11.0615) -> (27.578, -11.0615)
  line L142 (27.578, -11.0615) -> (27.578, -11.7939)
  line L143 (27.578, -11.7939) -> (26.9235, -11.7939)
  line L144 (20.5046, -12.9511) -> (24.0327, -12.9511)
  spline S87 degree 2 poles (24.0327, -12.9511) (23.9546, -12.3704) (23.5732, -12.0106) knots 0 0 0 1 1 1
  spline S88 degree 2 poles (23.5732, -12.0106) (23.1918, -11.6509) (22.598, -11.6509) knots 0 0 0 1 1 1
  spline S89 degree 2 poles (22.598, -11.6509) (21.7355, -11.6509) (21.2328, -12.3444) knots 0 0 0 1 1 1
  line L145 (21.2328, -12.3444) -> (20.5046, -12.0236)
  spline S90 degree 2 poles (20.5046, -12.0236) (20.86, -11.4732) (21.4278, -11.2045) knots 0 0 0 1 1 1
  spline S91 degree 2 poles (21.4278, -11.2045) (21.9956, -10.9401) (22.6154, -10.9401) knots 0 0 0 1 1 1
  spline S92 degree 2 poles (22.6154, -10.9401) (23.5776, -10.9401) (24.2623, -11.5382) knots 0 0 0 1 1 1
  spline S93 degree 2 poles (24.2623, -11.5382) (24.9428, -12.1407) (24.9428, -13.1592) knots 0 0 0 1 1 1
  spline S94 degree 2 poles (24.9428, -13.1592) (24.9428, -14.1257) (24.2797, -14.7498) knots 0 0 0 1 1 1
  spline S95 degree 2 poles (24.2797, -14.7498) (23.6122, -15.3739) (22.7497, -15.3739) knots 0 0 0 1 1 1
  spline S96 degree 2 poles (22.7497, -15.3739) (21.9046, -15.3739) (21.2198, -14.7628) knots 0 0 0 1 1 1
  spline S97 degree 2 poles (21.2198, -14.7628) (20.5306, -14.1561) (20.5046, -12.9511) knots 0 0 0 1 1 1
  spline S98 degree 2 poles (21.3541, -13.5493) (21.4408, -13.9913) (21.8136, -14.3467) knots 0 0 0 1 1 1
  spline S99 degree 2 poles (21.8136, -14.3467) (22.1863, -14.7065) (22.7281, -14.7065) knots 0 0 0 1 1 1
  spline S100 degree 2 poles (22.7281, -14.7065) (23.2222, -14.7065) (23.5732, -14.3814) knots 0 0 0 1 1 1
  spline S101 degree 2 poles (23.5732, -14.3814) (23.9243, -14.0607) (24.0023, -13.5493) knots 0 0 0 1 1 1
  line L146 (24.0023, -13.5493) -> (21.3541, -13.5493)
  line L147 (19.1264, -11.7939) -> (19.1264, -14.5244)
  line L148 (19.1264, -14.5244) -> (19.9715, -14.5244)
  line L149 (19.9715, -14.5244) -> (19.9715, -15.2569)
  line L150 (19.9715, -15.2569) -> (18.4676, -15.2569)
  line L151 (18.4676, -15.2569) -> (18.4676, -14.3121)
  spline S102 degree 2 poles (18.4676, -14.3121) (18.3289, -14.6805) (18.0819, -14.9232) knots 0 0 0 1 1 1
  spline S103 degree 2 poles (18.0819, -14.9232) (17.8348, -15.1659) (17.5618, -15.2439) knots 0 0 0 1 1 1
  spline S104 degree 2 poles (17.5618, -15.2439) (17.2844, -15.3219) (16.8076, -15.3219) knots 0 0 0 1 1 1
  line L152 (16.8076, -15.3219) -> (16.5909, -15.3219)
  line L153 (16.5909, -15.3219) -> (16.5909, -14.4898)
  line L154 (16.5909, -14.4898) -> (16.7556, -14.4898)
  spline S105 degree 2 poles (16.7556, -14.4898) (17.3841, -14.4898) (17.6961, -14.3641) knots 0 0 0 1 1 1
  spline S106 degree 2 poles (17.6961, -14.3641) (18.0038, -14.2384) (18.1555, -13.9047) knots 0 0 0 1 1 1
  spline S107 degree 2 poles (18.1555, -13.9047) (18.3029, -13.5753) (18.3029, -12.7171) knots 0 0 0 1 1 1
  line L155 (18.3029, -12.7171) -> (18.3029, -11.7939)
  line L156 (18.3029, -11.7939) -> (17.3884, -11.7939)
  line L157 (17.3884, -11.7939) -> (17.3884, -11.0615)
  line L158 (17.3884, -11.0615) -> (19.9716, -11.0615)
  line L159 (19.9716, -11.0615) -> (19.9716, -11.7939)
  line L160 (19.9716, -11.7939) -> (19.1264, -11.7939)
  line L161 (16.0925, -11.0615) -> (16.0925, -12.5004)
  line L162 (16.0925, -12.5004) -> (15.3557, -12.5004)
  line L163 (15.3557, -12.5004) -> (15.3557, -12.3617)
  spline S108 degree 2 poles (15.3557, -12.3617) (15.3167, -12.067) (15.0393, -11.8763) knots 0 0 0 1 1 1
  spline S109 degree 2 poles (15.0393, -11.8763) (14.7576, -11.6856) (14.3762, -11.6856) knots 0 0 0 1 1 1
  spline S110 degree 2 poles (14.3762, -11.6856) (13.9774, -11.6856) (13.739, -11.8243) knots 0 0 0 1 1 1
  spline S111 degree 2 poles (13.739, -11.8243) (13.5007, -11.963) (13.5007, -12.21) knots 0 0 0 1 1 1
  spline S112 degree 2 poles (13.5007, -12.21) (13.5007, -12.4484) (13.7, -12.5611) knots 0 0 0 1 1 1
  spline S113 degree 2 poles (13.7, -12.5611) (13.8951, -12.6738) (14.4802, -12.7691) knots 0 0 0 1 1 1
  spline S114 degree 2 poles (14.4802, -12.7691) (15.347, -12.9165) (15.7198, -13.2415) knots 0 0 0 1 1 1
  spline S115 degree 2 poles (15.7198, -13.2415) (16.0882, -13.5709) (16.0882, -14.091) knots 0 0 0 1 1 1
  spline S116 degree 2 poles (16.0882, -14.091) (16.0882, -14.6155) (15.6851, -14.9665) knots 0 0 0 1 1 1
  spline S117 degree 2 poles (15.6851, -14.9665) (15.282, -15.3219) (14.6232, -15.3219) knots 0 0 0 1 1 1
  spline S118 degree 2 poles (14.6232, -15.3219) (14.0294, -15.3219) (13.6004, -15.0792) knots 0 0 0 1 1 1
  line L164 (13.6004, -15.0792) -> (13.6004, -15.2569)
  line L165 (13.6004, -15.2569) -> (12.8679, -15.2569)
  line L166 (12.8679, -15.2569) -> (12.8679, -13.8657)
  line L167 (12.8679, -13.8657) -> (13.6004, -13.8657)
  line L168 (13.6004, -13.8657) -> (13.6004, -14.1214)
  spline S119 degree 2 poles (13.6004, -14.1214) (13.9341, -14.6371) (14.5712, -14.6371) knots 0 0 0 1 1 1
  spline S120 degree 2 poles (14.5712, -14.6371) (14.8963, -14.6371) (15.1086, -14.4941) knots 0 0 0 1 1 1
  spline S121 degree 2 poles (15.1086, -14.4941) (15.3167, -14.3554) (15.3167, -14.1214) knots 0 0 0 1 1 1
  spline S122 degree 2 poles (15.3167, -14.1214) (15.3167, -13.883) (15.126, -13.792) knots 0 0 0 1 1 1
  spline S123 degree 2 poles (15.126, -13.792) (14.9309, -13.7053) (14.2938, -13.6056) knots 0 0 0 1 1 1
  spline S124 degree 2 poles (14.2938, -13.6056) (13.6827, -13.5103) (13.3707, -13.3802) knots 0 0 0 1 1 1
  spline S125 degree 2 poles (13.3707, -13.3802) (13.0586, -13.2545) (12.8549, -12.9555) knots 0 0 0 1 1 1
  spline S126 degree 2 poles (12.8549, -12.9555) (12.6469, -12.6608) (12.6469, -12.2664) knots 0 0 0 1 1 1
  spline S127 degree 2 poles (12.6469, -12.2664) (12.6469, -11.6812) (13.0976, -11.3345) knots 0 0 0 1 1 1
  spline S128 degree 2 poles (13.0976, -11.3345) (13.544, -10.9921) (14.2592, -10.9921) knots 0 0 0 1 1 1
  spline S129 degree 2 poles (14.2592, -10.9921) (14.931, -10.9921) (15.3557, -11.2955) knots 0 0 0 1 1 1
  line L169 (15.3557, -11.2955) -> (15.3557, -11.0615)
  line L170 (15.3557, -11.0615) -> (16.0925, -11.0615)
  arc A7 (195, -107.5) -> (198, -110.5) centre (198, -107.5) ccw
  arc A8 (198, -103.5) -> (195, -106.5) centre (198, -106.5) ccw
  line L171 (105.5, -2.15) -> (105.5, -6)
  arc A9 (102.5, -9) -> (105.5, -6) centre (102.5, -6) ccw
  line L172 (102.5, -9) -> (101.5, -9)
  arc A10 (98.5, -6) -> (101.5, -9) centre (101.5, -6) ccw
  line L173 (98.5, -6) -> (98.5, -2.15)
  line L174 (98.5, -2.15) -> (3.15, -2.15)
  arc A11 (9, -106.5) -> (6, -103.5) centre (6, -106.5) ccw
  arc A12 (6, -110.5) -> (9, -107.5) centre (6, -107.5) ccw
  arc A13 (101.5, -195) -> (98.5, -198) centre (101.5, -198) ccw
  arc A14 (105.5, -198) -> (102.5, -195) centre (102.5, -198) ccw
extrude "Extrusion17" cut sketch "Skizze12" against normal blind 1 contours L19 L20 L21 L22 L23 L24 L25 S0 S1 S2 S3 S4 S5 S6 L26 L27 | L28 L29 L30 L31 L32 L33 L34 L35 L36 L37 L38 L39 L40 L41 L42 L43 L44 L45 | L46 L47 L48 L49 L50 L51 L52 L53 L54 L55 L56 L57 L58 L59 L60 L61 L62 L63 L64 L65 | S15 S16 S17 S18 S19 S20 S21 S22 | L66 L67 L68 L69 L70 L71 L72 L73 L74 L75 | L76 L77 S23 S24 S25 S26 S27 S28 S29 L78 S30 S31 S32 S33 S34 S35 L79 L80 | L81 L82 L83 L84 L85 L86 L87 L88 L89 L90 | L91 L92 L93 S36 S37 S38 S39 S40 S41 L94 S42 S43 S44 S45 L95 S46 S47 S48 S49 S50 L96 L97 | L99 L100 L101 S57 S58 S59 S60 S61 S62 S63 S64 S65 S66 S67 L102 L103 L104 L105 L106 S68 S69 S70 S71 S72 S73 S74 S75 S76 S77 S78 L107 L108 | L109 L110 L111 L112 L113 L114 L115 L116 L117 L118 L119 L120 L121 L122 L123 L124 L125 L126 L127 L128 L129 L130 L131 L132 L133 | S79 S80 S81 S82 S83 S84 S85 S86 | L134 L135 L136 L137 L138 L139 L140 L141 L142 L143 | L144 S87 S88 S89 L145 S90 S91 S92 S93 S94 S95 S96 S97 | L147 L148 L149 L150 L151 S102 S103 S104 L152 L153 L154 S105 S106 S107 L155 L156 L157 L158 L159 L160 | L161 L162 L163 S108 S109 S110 S111 S112 S113 S114 S115 S116 S117 S118 L164 L165 L166 L167 L168 S119 S120 S121 S122 S123 S124 S125 S126 S127 S128 S129 L169 L170
fillet "Abrundung7" radius 1.5 16 edges at (156.85, 22.15, 5.125) (153.85, 22.15, 5.125) (117.5497, 150, 5.125) (86.4503, 150, 5.125) (173.85, 136.85, 5.125) (176.85, 136.85, 5.125) (176.85, 181.85, 5.125) (173.85, 181.85, 5.125) (104.8831, 188, 5.125) (99.117, 188, 5.125) (35.15, 181.85, 5.125) (32.15, 181.85, 5.125) (35.15, 22.15, 5.125) (156.85, 67.15, 5.125) (153.85, 67.15, 5.125) (32.15, 22.15, 5.125)